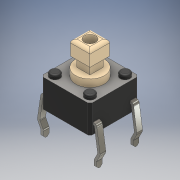
# Autodesk Inventor part: 49-0005
Saved by Autodesk Inventor 2018 (Build 220112000, 112)
## iProperties
Created: 2019-09-25
Part Number: 49-0005
Material: ABS Plastic
Document SubType Name: Modeling
Designer: Bradley
Density: 1.06 g/cm^3
Appearance: Smooth - Black
Author: Bradley
Autodesk Inventor part; units mm, degrees
ref_plane "YZ Plane" through (0, 0, 0) normal (1, 0, 0) x (0, 1, 0)
ref_plane "XZ Plane" through (0, 0, 0) normal (0, 1, 0) x (-1, 0, 0)
ref_plane "XY Plane" through (0, 0, 0) normal (0, 0, 1) x (1, 0, 0)
sketch "Sketch1" plane through (0, 0, 0) normal (0, 0, 1) x (1, 0, 0)
  line L0 (-2.75, -3) -> (2.75, -3)
  line L1 (3, -2.75) -> (3, 2.75)
  line L2 (2.75, 3) -> (-2.75, 3)
  line L3 (-3, 2.75) -> (-3, -2.75)
  line L4 (-3, -3) -> (3, 3) construction
  line L5 (3, -3) -> (-3, 3) construction
  line L6 (-2.75, 3) -> (-3, 2.75)
  line L7 (-3, -2.75) -> (-2.75, -3)
  line L8 (2.75, -3) -> (3, -2.75)
  line L9 (3, 2.75) -> (2.75, 3)
  point P0 (0, 0)
  dimension "d0" = 6
  dimension "d1" = 0.25
  dimension "d2" = 0.25
  dimension "d3" = 0.25
  dimension "d4" = 0.25
  dimension "d5" = 0.25
  dimension "d6" = 0.25
  dimension "d7" = 0.25
  dimension "d8" = 0.25
  constraints: 20 end point, 8 point on line, 2 midpoint, 2 parallel, 2 perpendicular, 1 horizontal
  measures "d0" distance of L5.end L4.end
  measures "d1" distance of L2.end L5.end
  measures "d2" distance of L3.start L5.end
  measures "d3" distance of L3.end L4.start
  measures "d4" distance of L0.start L4.start
  measures "d5" distance of L0.end L5.start
  measures "d6" distance of L1.start L5.start
  measures "d7" distance of L1.end L4.end
  measures "d8" distance of L2.start L4.end
extrude "Extrusion1" add sketch "Sketch1" along normal mid plane 3.4
sketch "Sketch2" plane through (0, 0, 1.7) normal (0, 0, 1) x (1, 0, 0)
  line L0 (-2.15, -2.15) -> (2.15, -2.15) construction
  line L1 (2.15, -2.15) -> (2.15, 2.15) construction
  line L2 (2.15, 2.15) -> (-2.15, 2.15) construction
  line L3 (-2.15, 2.15) -> (-2.15, -2.15) construction
  line L4 (-2.15, -2.15) -> (2.15, 2.15) construction
  line L5 (2.15, -2.15) -> (-2.15, 2.15) construction
  circle A0 centre (-2.15, 2.15) radius 0.6
  circle A1 centre (2.15, 2.15) radius 0.6
  circle A2 centre (2.15, -2.15) radius 0.6
  circle A3 centre (-2.15, -2.15) radius 0.6
  point P0 (0, 0)
  dimension "d11" = 4.3
  dimension "d12" = 1.2
  constraints: 12 end point, 4 centre point, 4 coincident, 3 equal radius, 2 midpoint, 2 parallel, 2 perpendicular, 1 horizontal
  measures "d11" distance of L1.end L2.end
  measures "d12" diameter of A0
extrude "Extrusion2" add sketch "Sketch2" along normal blind 0.5
sketch "Sketch3" plane through (0, 0, 1.7) normal (0, 0, 1) x (1, 0, 0)
  circle A0 centre (0, 0) radius 1.75
  dimension "d15" = 3.5
  constraints: 1 centre point, 1 coincident
  measures "d15" diameter of A0
extrude "Extrusion3" add sketch "Sketch3" along normal blind 0.9
sketch "Sketch4" plane through (0, 0, 2.6) normal (0, 0, 1) x (1, 0, 0)
  line L0 (-0.8, -0.8) -> (0.8, -0.8)
  line L1 (0.8, -0.8) -> (0.8, 0.8)
  line L2 (0.8, 0.8) -> (-0.8, 0.8)
  line L3 (-0.8, 0.8) -> (-0.8, -0.8)
  line L4 (-0.8, -0.8) -> (0.8, 0.8) construction
  line L5 (0.8, -0.8) -> (-0.8, 0.8) construction
  point P0 (0, 0)
  dimension "d18" = 1.6
  constraints: 12 end point, 2 midpoint, 2 parallel, 2 perpendicular, 1 horizontal
  measures "d18" distance of L2.end L1.end
extrude "Extrusion4" add sketch "Sketch4" along normal blind 1.2
sketch "Sketch5" plane through (0, 0, 3.8) normal (0, 0, 1) x (1, 0, 0)
  circle A0 centre (0, 0) radius 0.7
  line L0 (-1.2, -1.2) -> (1.2, -1.2)
  line L1 (1.2, -1.2) -> (1.2, 1.2)
  line L2 (1.2, 1.2) -> (-1.2, 1.2)
  line L3 (-1.2, 1.2) -> (-1.2, -1.2)
  line L4 (-1.2, -1.2) -> (1.2, 1.2) construction
  line L5 (1.2, -1.2) -> (-1.2, 1.2) construction
  dimension "d21" = 1.4
  dimension "d22" = 2.4
  constraints: 12 end point, 2 midpoint, 2 parallel, 2 perpendicular, 1 centre point, 1 coincident, 1 horizontal
  measures "d21" diameter of A0
  measures "d22" distance of L2.end L1.end
extrude "Extrusion5" add sketch "Sketch5" along normal blind 1.8
fillet "Fillet1" radius 0.4 4 edges at (0, 1.2, 5.6) (-1.2, 0, 5.6) (0, -1.2, 5.6) (1.2, 0, 5.6)
sketch "Sketch6" plane through (0, 0, 0) normal (0, 1, 0) x (-1, 0, 0)
  line L0 (-3, -1.7) -> (-3, 1.7) projected
  line L1 (-3, -1.7) -> (-3, 1.7) projected
  line L2 (-3.1484, -0.828) -> (-3.5321, -3.4214)
  arc A0 (-3.5321, -3.4214) -> (-3.5173, -3.5117) centre (-3.3838, -3.4434) ccw
  line L3 (-3.5173, -3.5117) -> (-3.1493, -4.2312)
  arc A1 (-3.1, -4.4361) -> (-3.1493, -4.2312) centre (-3.55, -4.4361) ccw
  line L4 (-3.1, -4.4361) -> (-3.1, -5.2)
  line L5 (-3.1, -5.2) -> (-3.4, -5.2)
  line L6 (-3.4, -5.2) -> (-3.4, -4.4361)
  arc A2 (-3.4, -4.4361) -> (-3.4164, -4.3678) centre (-3.55, -4.4361) ccw
  line L7 (-3.4164, -4.3678) -> (-3.7844, -3.6483)
  arc A3 (-3.8289, -3.3775) -> (-3.7844, -3.6483) centre (-3.3838, -3.4434) ccw
  line L8 (-3.8289, -3.3775) -> (-3.4452, -0.7841)
  line L9 (-3.8289, -3.3775) -> (-3.85, -3.52) construction
  line L10 (-3.85, -3.52) -> (-3.7844, -3.6483) construction
  line L11 (-3.4, -4.4361) -> (-3.4, -4.4) construction
  line L12 (-3.4, -4.4) -> (-3.4164, -4.3678) construction
  arc A4 (-3, -0.7) -> (-3.1484, -0.828) centre (-3, -0.85) ccw
  arc A5 (-3, -0.4) -> (-3.4452, -0.7841) centre (-3, -0.85) ccw
  line L13 (2.75, -1.7) -> (-2.75, -1.7) projected
  line L14 (0, 0) -> (0, -1.7) construction
  line L15 (-3, -0.4) -> (-3, -0.7)
  line L16 (3.1484, -0.828) -> (3.5321, -3.4214)
  arc A6 (3.5173, -3.5117) -> (3.5321, -3.4214) centre (3.3838, -3.4434) ccw
  line L17 (3.5173, -3.5117) -> (3.1493, -4.2312)
  arc A7 (3.1493, -4.2312) -> (3.1, -4.4361) centre (3.55, -4.4361) ccw
  line L18 (3.1, -4.4361) -> (3.1, -5.2)
  line L19 (3.1, -5.2) -> (3.4, -5.2)
  line L20 (3.4, -5.2) -> (3.4, -4.4361)
  arc A8 (3.4164, -4.3678) -> (3.4, -4.4361) centre (3.55, -4.4361) ccw
  line L21 (3.4164, -4.3678) -> (3.7844, -3.6483)
  arc A9 (3.7844, -3.6483) -> (3.8289, -3.3775) centre (3.3838, -3.4434) ccw
  line L22 (3.8289, -3.3775) -> (3.4452, -0.7841)
  line L23 (3.8289, -3.3775) -> (3.85, -3.52) construction
  line L24 (3.85, -3.52) -> (3.7844, -3.6483) construction
  line L25 (3.4, -4.4361) -> (3.4, -4.4) construction
  line L26 (3.4, -4.4) -> (3.4164, -4.3678) construction
  arc A10 (3.1484, -0.828) -> (3, -0.7) centre (3, -0.85) ccw
  arc A11 (3.4452, -0.7841) -> (3, -0.4) centre (3, -0.85) ccw
  line L27 (3, -0.4) -> (3, -0.7)
  dimension "d26" = 0.3
  dimension "d28" = 3.5
  dimension "d29" = 3.4
  dimension "d30" = 0.15
  dimension "d31" = 3.85
  dimension "d32" = 1.82
  dimension "d33" = 0.8
  dimension "d34" = 1
  constraints: 50 end point, 24 point on circle, 22 symmetric about line, 12 centre point, 12 tangent, 4 collinear, 3 concentric, 3 point on line, 2 equal radius, 2 parallel, 2 perpendicular, 2 vertical, 1 midpoint, 6 other
  measures "d26" distance of L4.end L5.end
  measures "d28" distance from line of L5 L0.start
  measures "d29" distance from line of L6 L14.start
  measures "d30" radius of A2
  measures "d31" horizontal distance of L14.start L9.end
  measures "d32" vertical distance of L9.end L0.start
  measures "d33" distance from line of L5 L11.end
  measures "d34" distance of L0.start L15.end
extrude "Extrusion6" add sketch "Sketch6" along normal mid plane 5.2
sketch "Sketch7" plane through (0, 0, 0) normal (0, 0, 1) x (1, 0, 0)
  line L0 (-3, 2.75) -> (-3, -2.75) projected
  line L1 (-4, 1.9) -> (-3, 1.9)
  line L2 (-3, 1.9) -> (-3, -1.9)
  line L3 (-3, -1.9) -> (-4, -1.9)
  line L4 (-4, -1.9) -> (-4, 1.9)
  line L5 (3, -2.75) -> (3, 2.75) projected
  line L6 (4, 1.9) -> (3, 1.9)
  line L7 (3, 1.9) -> (3, -1.9)
  line L8 (3, -1.9) -> (4, -1.9)
  line L9 (4, -1.9) -> (4, 1.9)
  point P0 (0, 0)
  point P1 (-3.8289, 2.6)
  point P2 (3, 0)
  point P3 (3, 0)
  point P4 (-3, 0)
  dimension "d37" = 0.7
  dimension "d40" = 1
  constraints: 16 end point, 6 midpoint, 4 parallel, 3 point on line, 2 horizontal, 2 perpendicular, 1 collinear
  measures "d37" distance from line of point (-3.829, 2.6) L1
  measures "d40" distance of L1.start L1.end
extrude "Extrusion7" cut sketch "Sketch7" against normal through all
chamfer "Chamfer1" distance 0.25 angle 45 8 edges at (-3.25, -2.6, -5.2) (-3.25, -1.9, -5.2) (3.25, -2.6, -5.2) (3.25, -1.9, -5.2) (3.25, 1.9, -5.2) (3.25, 2.6, -5.2) (-3.25, 1.9, -5.2) (-3.25, 2.6, -5.2)
fillet "Fillet2" radius 0.2 4 edges at (-2.75, -2.15, 2.2) (1.55, -2.15, 2.2) (-2.75, 2.15, 2.2) (1.55, 2.15, 2.2)
equation "\"d2\" = d1"
equation "\"d3\" = d1"
equation "\"d4\" = d3"
equation "\"d5\" = d1"
equation "\"d6\" = d5"
equation "\"d7\" = d1"
equation "\"d8\" = d7"
equation "\"d30\" = 0.5 * d26"
body "Solid1"
